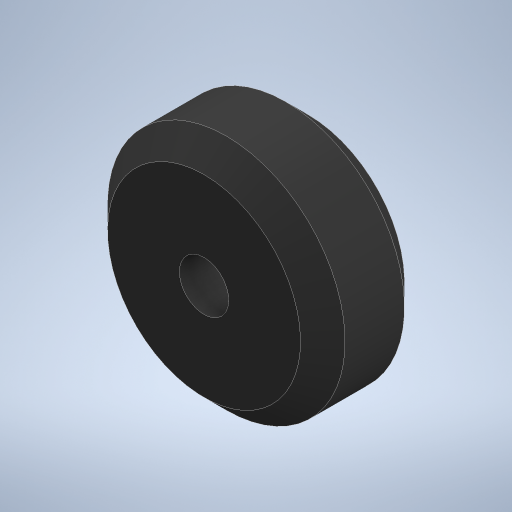
# Autodesk Inventor part: VSlot RollerWheel
Saved by Autodesk Inventor 2023 (Build 270158000, 158)
## iProperties
Created: 2023-04-10
Part Number: VSlot RollerWheel
Material: Rubber
Document SubType Name: Modeling
Designer: ethan
Density: 0.93 g/cm^3
Appearance: Rubber - Black
Author: ethan
Autodesk Inventor part; units mm, degrees
ref_plane "YZ Plane" through (0, 0, 0) normal (1, 0, 0) x (0, 1, 0)
ref_plane "XZ Plane" through (0, 0, 0) normal (0, 1, 0) x (-1, 0, 0)
ref_plane "XY Plane" through (0, 0, 0) normal (0, 0, 1) x (1, 0, 0)
sketch "Sketch1" plane through (0, 0, 0) normal (1, 0, 0) x (0, 1, 0)
  circle A0 centre (0, 0) radius 2.15 construction
  line L0 (2.8308, 3.75) -> (-2.8308, 3.75) construction
  line L1 (-2.8308, 3.75) -> (-5.5, 6.4192) construction
  line L2 (-5.5, 6.4192) -> (-5.5, 8.2) construction
  line L3 (-5.5, 8.2) -> (-3.6328, 8.2) construction
  arc A1 (-3.6328, 8.2) -> (-3.4914, 8.5414) centre (-3.6328, 8.4) ccw construction
  line L4 (-3.4914, 8.5414) -> (-4.95, 10) construction
  line L5 (-4.95, 10) -> (-10, 10) construction
  line L6 (-10, 10) -> (-10, 4.95) construction
  line L7 (-10, 4.95) -> (-8.5414, 3.4914) construction
  arc A2 (-8.5414, 3.4914) -> (-8.2, 3.6328) centre (-8.4, 3.6328) ccw construction
  line L8 (-8.2, 3.6328) -> (-8.2, 5.5) construction
  line L9 (-8.2, 5.5) -> (-6.4192, 5.5) construction
  line L10 (-6.4192, 5.5) -> (-3.75, 2.8308) construction
  line L11 (-3.75, 2.8308) -> (-3.75, -2.8308) construction
  line L12 (-3.75, -2.8308) -> (-6.4192, -5.5) construction
  line L13 (-6.4192, -5.5) -> (-8.2, -5.5) construction
  line L14 (-8.2, -5.5) -> (-8.2, -3.6328) construction
  arc A3 (-8.2, -3.6328) -> (-8.5414, -3.4914) centre (-8.4, -3.6328) ccw construction
  line L15 (-8.5414, -3.4914) -> (-10, -4.95) construction
  line L16 (-10, -4.95) -> (-10, -10) construction
  line L17 (-10, -10) -> (-4.95, -10) construction
  line L18 (-4.95, -10) -> (-3.4914, -8.5414) construction
  arc A4 (-3.4914, -8.5414) -> (-3.6328, -8.2) centre (-3.6328, -8.4) ccw construction
  line L19 (-3.6328, -8.2) -> (-5.5, -8.2) construction
  line L20 (-5.5, -8.2) -> (-5.5, -6.4192) construction
  line L21 (-5.5, -6.4192) -> (-2.8308, -3.75) construction
  line L22 (-2.8308, -3.75) -> (2.8308, -3.75) construction
  line L23 (2.8308, -3.75) -> (5.5, -6.4192) construction
  line L24 (5.5, -6.4192) -> (5.5, -8.2) construction
  line L25 (5.5, -8.2) -> (3.6328, -8.2) construction
  arc A5 (3.6328, -8.2) -> (3.4914, -8.5414) centre (3.6328, -8.4) ccw construction
  line L26 (3.4914, -8.5414) -> (4.95, -10) construction
  line L27 (4.95, -10) -> (10, -10) construction
  line L28 (10, -10) -> (10, -4.95) construction
  line L29 (10, -4.95) -> (8.5414, -3.4914)
  arc A6 (8.5414, -3.4914) -> (8.2, -3.6328) centre (8.4, -3.6328) ccw construction
  line L30 (8.2, -3.6328) -> (8.2, -5.5) construction
  line L31 (8.2, -5.5) -> (6.4192, -5.5) construction
  line L32 (6.4192, -5.5) -> (3.75, -2.8308) construction
  line L33 (3.75, -2.8308) -> (3.75, 2.8308) construction
  line L34 (3.75, 2.8308) -> (6.4192, 5.5) construction
  line L35 (6.4192, 5.5) -> (8.2, 5.5) construction
  line L36 (8.2, 5.5) -> (8.2, 3.6328) construction
  arc A7 (8.2, 3.6328) -> (8.5414, 3.4914) centre (8.4, 3.6328) ccw construction
  line L37 (8.5414, 3.4914) -> (10, 4.95)
  line L38 (10, 4.95) -> (10, 10) construction
  line L39 (10, 10) -> (4.95, 10) construction
  line L40 (4.95, 10) -> (3.4914, 8.5414) construction
  arc A8 (3.4914, 8.5414) -> (3.6328, 8.2) centre (3.6328, 8.4) ccw construction
  line L41 (3.6328, 8.2) -> (5.5, 8.2) construction
  line L42 (5.5, 8.2) -> (5.5, 6.4192) construction
  line L43 (5.5, 6.4192) -> (2.8308, 3.75) construction
  line L44 (10.3, 5.25) -> (10.3, -5.25) construction
  line L45 (10, 4.95) -> (10.3, 5.25)
  line L46 (10, -4.95) -> (10.3, -5.25)
  line L47 (8.05, 3) -> (8.05, -3)
  line L48 (8.5414, 3.4914) -> (8.05, 3)
  line L49 (8.5414, -3.4914) -> (8.05, -3)
  line L50 (32.05, 3) -> (32.05, -3)
  line L51 (10.3, 5.25) -> (29.8, 5.25)
  line L52 (10.3, -5.25) -> (29.8, -5.25)
  line L53 (29.8, 5.25) -> (32.05, 3)
  line L54 (32.05, -3) -> (29.8, -5.25)
  line L55 (20.05, 5.25) -> (20.05, -5.25) construction
  line L56 (22.55, 5.25) -> (22.55, -5.25)
  line L57 (17.55, 5.25) -> (17.55, -5.25)
  dimension "d0" = 10.5
  dimension "d1" = 45
  dimension "d2" = 6
  dimension "d3" = 6
  dimension "d4" = 24
  dimension "d5" = 135
  dimension "d7" = 2.5
  dimension "d8" = 2.5
  constraints: 116 end point, 17 vertical, 16 horizontal, 16 point on circle, 9 centre point, 3 perpendicular, 3 point on line, 2 midpoint, 1 collinear, 1 parallel, 1 tangent, 88 other
  measures "d0" distance of L44.start L44.end
  measures "d1" angle of L28 L46
  measures "d2" distance of L47.start L47.end
  measures "d3" distance of L50.start L50.end
  measures "d4" distance between parallel lines of L47 L50
  measures "d5" angle of L51 L53
  measures "d7" distance from line of L55.start L57
  measures "d8" distance from line of L55.start L56
revolve "Revolution1" add sketch "Sketch1" angle 360 about axis through (0, 20.05, 5.25) along (0, 0, -1) contours L56 L51 L53 L50 L54 L52
body "Solid1"
